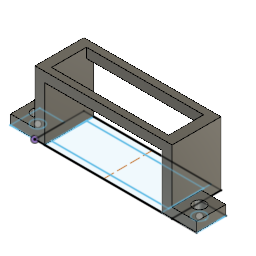
OdPowerStrap v4 (Autodesk Fusion 360 design; units mm, degrees)
Autodesk Fusion 360 part; units mm, degrees
sketch "Sketch1" plane through (0, 0, 0) normal (0, 0, 1) x (1, 0, 0)
  line L0 (0, 0) -> (28, 0)
  line L1 (28, 0) -> (28, 10)
  line L2 (28, 10) -> (0, 10)
  line L3 (0, 10) -> (0, 0)
  line L4 (2, 0) -> (25.8784, 0)
  line L5 (25.8784, 0) -> (25.8784, 10)
  line L6 (25.8784, 10) -> (2, 10)
  line L7 (2, 10) -> (2, 0)
  line L8 (-5, 0) -> (0, 0)
  line L9 (0, 0) -> (0, 6)
  line L10 (0, 6) -> (-5, 6)
  line L11 (-5, 6) -> (-5, 0)
  line L12 (28, 6) -> (33, 6)
  line L13 (33, 6) -> (33, 0)
  line L14 (33, 0) -> (28, 0)
  line L15 (28, 0) -> (28, 6)
  circle A0 centre (-2.4098, 3) radius 1.2381
  line L16 (13.9392, 10) -> (14, 0) construction
  line L17 (2, 8.5375) -> (25.8784, 8.5375)
  line L18 (25.8784, 8.5375) -> (25.8784, 1.4031)
  line L19 (25.8784, 1.4031) -> (2, 1.4031)
  line L20 (2, 1.4031) -> (2, 8.5375)
  circle A1 centre (30.3721, 3.1993) radius 1.2381
  dimension "d1" = 28
  dimension "d2" = 10
  dimension "d11" = 6
  dimension "d12" = 3
  dimension "d14" = 6
  constraint horizontal L0
  constraint vertical L1
  constraint horizontal L2
  constraint vertical L3
  constraint coincident L0.start L3.end
  constraint horizontal L4
  constraint vertical L5
  constraint horizontal L6
  constraint vertical L7
  constraint coincident L2 L5.end
  constraint coincident L0 L4.start
  constraint horizontal L8
  constraint vertical L9
  constraint horizontal L10
  constraint vertical L11
  constraint coincident L3 L9.end
  constraint horizontal L12
  constraint vertical L13
  constraint horizontal L14
  constraint vertical L15
  constraint coincident L1 L12.start
  constraint midpoint L6 L16.start
  constraint midpoint L0 L16.end
  constraint horizontal L17
  constraint vertical L18
  constraint horizontal L19
  constraint vertical L20
  constraint coincident L5 L18.end
  constraint coincident L7 L17.start
  constraint coincident L0.end L1.start
  constraint symmetric A0 L16 A1
  measures "d1" distance of L0.start L0.end
  measures "d2" distance of L0.start L2.end
  measures "d11" distance of L8.start L10.end
  measures "d12" distance of L8 A0.centre
  measures "d14" distance of L12.start L0.end
extrude "Extrude1" add sketch "Sketch1" along normal blind 2 contours L3 L8 L9 L10 L11 | L1 L12 L13 L14 L15 makes body 1 at (-2.5008, 0.5884, 0) makes body 2 at (30.4882, 0.6549, 0)
extrude "Extrude2" add sketch "Sketch1" along normal blind 13 contours L0 L2 L3 L7 L9 L20 | L0 L4 L5 L7 L19 | L0 L1 L2 L5 L15 L18 | L2 L5 L6 L7 L17 bodies 1 2
extrude "Extrude3" cut sketch "Sketch1" along normal blind 11 contours L0 L4 L5 L7 L19 | L5 L7 L17 L18 L19 L20 | L2 L5 L6 L7 L17 bodies 1
